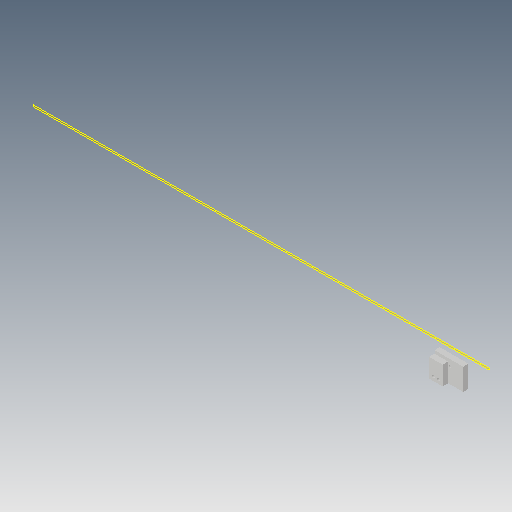
# Autodesk Inventor part: RollerSupport
Saved by Autodesk Inventor 2018 (Build 220112000, 112)
## iProperties
Created: 2018-11-28
Part Number: RollerSupport
Material: Generic
Document SubType Name: Modeling
Designer: ball
Density: 1 g/cm^3
Appearance: Default
Author: ball
Autodesk Inventor part; units mm, degrees
ref_plane "YZ Plane" through (0, 0, 0) normal (1, 0, 0) x (0, 1, 0)
ref_plane "XZ Plane" through (0, 0, 0) normal (0, 1, 0) x (-1, 0, 0)
ref_plane "Work Plane1" through (0, 0, 0) normal (0, 0, 1) x (1, 0, 0)
ref_plane "Work Plane2" through (-55.1754, -24.0887, 15.745) normal (0, 0, -1) x (0, 1, 0)
sketch "Sketch1" plane through (0, 0, 0) normal (0, 0, 1) x (1, 0, 0)
  line L0 (-15.577, -32.8319) -> (-625.177, -32.8319)
  line L1 (-15.577, -13.7819) -> (-625.177, -13.7819)
  line L2 (-51.9475, -0.5269) -> (-51.9475, -17.8187)
  line L3 (-15.577, -10.6107) -> (-15.577, -36.0031)
  line L4 (-51.9475, -45.8894) -> (-31.9475, -45.8894)
  line L5 (-51.9475, -13.7819) -> (-9.7581, -13.7819)
  line L6 (-9.7581, -13.7819) -> (-9.7581, -45.8894)
  line L7 (-9.7581, -45.8894) -> (-51.9475, -45.8894)
  line L8 (-51.9475, -45.8894) -> (-51.9475, -13.7819)
  arc A0 (-55.86, -21.5601) -> (-54.5757, -21.9771) centre (-55.7173, -23.3069) ccw
  arc A1 (-28.9193, -21.5601) -> (-27.635, -21.9771) centre (-28.7766, -23.3069) ccw
  circle A2 centre (-55.7173, -23.3069) radius 1.778
  circle A3 centre (-28.7766, -23.3069) radius 1.778
  circle A4 centre (-37.9475, -17.22) radius 2
  circle A5 centre (-37.9475, -17.22) radius 2
  point P0 (0, 0)
extrude "Extrusion1" add sketch "Sketch1" along normal up to surface (15.745 mm away) contours L3 L5 L6 L7 L4 L8 L0 | L0 L8 L2 L1 L3 | A4
sketch "Sketch2" plane through (-51.9475, -13.7819, 15.745) normal (0, 0, 1) x (1, 0, 0)
  circle A0 centre (6, -26.745) radius 2 projected
  circle A1 centre (14, -26.745) radius 2 projected
  circle A2 centre (6, -26.745) radius 2
  circle A3 centre (14, -26.745) radius 2
  point P0 (51.9475, 13.7819)
  constraints: 2 centre point, 2 coincident, 2 concentric
hole "Hole1" at (-45.9475, -40.5269, 15.745) direction (0, 0, -1) diameter 3.9878 end through all
sketch "Sketch3" plane through (-51.9475, -13.7819, 15.745) normal (0, 0, 1) x (1, 0, 0)
  circle A0 centre (14, -26.745) radius 2 projected
  circle A1 centre (14, -26.745) radius 2
  point P0 (51.9475, 13.7819)
  constraints: 1 centre point, 1 coincident, 1 concentric
hole "Hole2" at (-37.9475, -40.5269, 15.745) direction (0, 0, -1) diameter 3.9878 end through all
sketch "Sketch5" plane through (-51.9475, -13.7819, 15.745) normal (0, 0, 1) x (1, 0, 0)
  arc A0 (5.0711, -20.6445) -> (7.8995, -17.8161) centre (6.4853, -19.2303) ccw projected
  line L0 (4.5858, -20.1592) -> (5.0711, -20.6445) projected
  arc A1 (7.4142, -17.3308) -> (4.5858, -20.1592) centre (6, -18.745) ccw projected
  line L1 (7.8995, -17.8161) -> (7.4142, -17.3308) projected
  arc A2 (7.8995, -3.6739) -> (5.0711, -0.8455) centre (6.4853, -2.2597) ccw projected
  line L2 (7.4142, -4.1592) -> (7.8995, -3.6739) projected
  arc A3 (4.5858, -1.3308) -> (7.4142, -4.1592) centre (6, -2.745) ccw projected
  line L3 (5.0711, -0.8455) -> (4.5858, -1.3308) projected
  circle A4 centre (6, -26.745) radius 2 projected
  circle A5 centre (14, -26.745) radius 2 projected
  line L4 (20, -4.0368) -> (20, 13.255) projected
  line L5 (0, 13.255) -> (20, 13.255) projected
  line L6 (0, 13.255) -> (0, -4.0368) projected
  arc A6 (0, -17.4532) -> (0, -4.0368) centre (-2, -10.745) ccw projected
  line L7 (0, -17.4532) -> (0, -32.1075) projected
  line L8 (0, -32.1075) -> (20, -32.1075) projected
  line L9 (20, -32.1075) -> (20, -17.4532) projected
  arc A7 (20, -4.0368) -> (20, -17.4532) centre (22, -10.745) ccw projected
  circle A8 centre (6, 5.255) radius 2 projected
  circle A9 centre (14, 5.255) radius 2 projected
  arc A10 (12.1005, -17.8161) -> (14.9289, -20.6445) centre (13.5147, -19.2303) ccw projected
  line L10 (12.5858, -17.3308) -> (12.1005, -17.8161) projected
  arc A11 (15.4142, -20.1592) -> (12.5858, -17.3308) centre (14, -18.745) ccw projected
  line L11 (14.9289, -20.6445) -> (15.4142, -20.1592) projected
  line L12 (10.6863, -8.745) -> (9.3137, -8.745) projected
  arc A12 (10.6863, -12.745) -> (10.6863, -8.745) centre (10.6863, -10.745) ccw projected
  line L13 (9.3137, -12.745) -> (10.6863, -12.745) projected
  arc A13 (9.3137, -8.745) -> (9.3137, -12.745) centre (9.3137, -10.745) ccw projected
  arc A14 (14.9289, -0.8455) -> (12.1005, -3.6739) centre (13.5147, -2.2597) ccw projected
  line L14 (15.4142, -1.3308) -> (14.9289, -0.8455) projected
  arc A15 (12.5858, -4.1592) -> (15.4142, -1.3308) centre (14, -2.745) ccw projected
  line L15 (12.1005, -3.6739) -> (12.5858, -4.1592) projected
  line L16 (0, -32.1075) -> (42.1894, -32.1075) projected
  line L17 (42.1894, 0) -> (0, 0) projected
  line L18 (42.1894, -32.1075) -> (20, -32.1075)
  line L19 (20, -32.1075) -> (20, 0)
  line L20 (20, 0) -> (42.1894, 0)
  line L21 (42.1894, 0) -> (42.1894, -32.1075)
  point P0 (51.9475, 13.7819)
  constraints: 8 end point, 2 parallel, 2 point on line, 1 horizontal, 1 perpendicular
extrude "Extrusion2" cut sketch "Sketch5" against normal blind 8.0264 contours L4 L17 L21 L16 L9 L19
sketch "Sketch7" plane through (-51.9475, -13.7819, 0) normal (0, 1, 0) x (1, 0, 0)
  line L0 (20, -15.745) -> (20, -7.7186) projected
  line L1 (0, 0) -> (0, -15.745) projected
  line L2 (20, -15.745) -> (0, -15.745)
  line L3 (0, -15.745) -> (0, -7.7186)
  line L4 (0, -7.7186) -> (20, -7.7186)
  line L5 (20, -7.7186) -> (20, -15.745)
  point P0 (51.9475, 0)
  dimension "d35" = 8.0264
  constraints: 8 end point, 2 parallel, 1 horizontal, 1 perpendicular, 1 point on line
  measures "d35" distance of L2.end L3.end
extrude "Extrusion3" cut sketch "Sketch7" against normal blind 4.445
body "Solid1"
